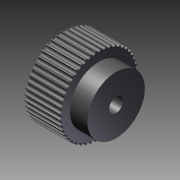
# Autodesk Inventor part: zrr_htd_3m15_8_17034800
Saved by Autodesk Inventor 2011 SP1 (Build 150282100, 282)
## iProperties
Created: 2018-07-07
Part Number: zrr_htd_3m15_8_17034800
Catalog Web Link: www.cadenas.de
Description: zrr_htd_3m15-HTD Pulleys Profile 3M, Timing Belt Width 15mm
Vendor: MAEDLER
Document SubType Name: Modeling
Designer: psAdmin
Manufacturer: MAEDLER
Mass: 101 g
Surface Area: 87.5363 cm^2
Volume: 36.8205 cm^3
Density: 1 g/cm^3
Category: PARTsolutions
Company: MAEDLER
Title: zrr_htd_3m15_8_17034800
Author: Cadenas PARTsolutions
Comments: HTD Pulleys Profile 3M, Timing Belt Width 15mm
PSOL_IDENT_0: {$CADENAS_DATA\23d-libs\maedler\antriebselemente\zahnriemenraeder_zahnriemen\zahnriemenraeder\htd-pr
PSOL_IDENT_1: ofil\zrr_htd_3m15.prj},197 {VTYP=3D},{NB=zrr_htd_3m15_8_17034800},{LINA=zrr_htd_3m15_8_17034800},{NN=
PSOL_IDENT_2: zrr_htd_3m15},{DATE=16.06.2017 10:47:49},{GEOMDATE=09.06.2016 09:07:07},{VERSION=},{LINEID=380},{LIN
PSOL_IDENT_3: ESUBID=-1},{WBVAR=BX}  {NB=zrr_htd_3m15_8_17034800},{LINA=zrr_htd_3m15_8_17034800},{KT=DUMMY},{ARTNR=
PSOL_IDENT_4: 17034800},{PDF=PDF Katalogseite},{AUSF=48-3M-15-2},{MAT=Aluminium},{ZTL=3.000},{ZRB=15.000},{Z=48.00
PSOL_IDENT_5: 0},{AUS=2},{ZS=45.080},{BS=0.000},{DO=45.840},{ND=33.000},{B=20.000},{L=30.000},{I=0.000},{VB=8.000}
PSOL_IDENT_6: ,{FB=20.000},{BX=8},{GEW=101.000},{ZT=1.200},{ZB=1.800},{T=2.000},{BB=1.000}
NN: zrr_htd_3m15
NT: HTD-Zahnriemenräder Profil 3M, Zahnriemenbreite 15mm
NB: zrr_htd_3m15_8_17034800
NBSYN: zrr_htd_3m15_$BX._$ARTNR.
LINA: zrr_htd_3m15_8_17034800
ARTNR: 17034800
PDF: PDF Katalogseite
AUSF: 48-3M-15-2
MAT: Aluminium
ZTL: 3.000
ZRB: 15.000
Z: 48.000
AUS: 2
ZS: 45.080
BS: 0.000
DO: 45.840
ND: 33.000
B: 20.000
L: 30.000
I: 0.000
VB: 8.000
FB: 20.000
BX: 8
GEW: 101.000
ZT: 1.200
ZB: 1.800
T: 2.000
BB: 1.000
SUPPLIER: MAEDLER
ARTICLENO: zrr_htd_3m15_8_17034800
BOMINFO: zrr_htd_3m15_8_17034800
CREATOR: CADENAS GmbH
Autodesk Inventor part; units mm, degrees
ref_plane "YZ Plane" through (0, 0, 0) normal (1, 0, 0) x (0, 1, 0)
ref_plane "XZ Plane" through (0, 0, 0) normal (0, 1, 0) x (-1, 0, 0)
ref_plane "XY Plane" through (0, 0, 0) normal (0, 0, 1) x (1, 0, 0)
sketch "Sketch_5" plane through (0, 0, 0) normal (0, 0, 1) x (1, 0, 0)
  line L0 (500, 0) -> (-500, 0)
  line L1 (0, 0) -> (0, 22.54)
  line L2 (0, 22.54) -> (20, 22.54)
  line L3 (20, 22.54) -> (20, 16.5)
  line L4 (20, 16.5) -> (30, 16.5)
  line L5 (30, 16.5) -> (30, 0)
  line L6 (30, 0) -> (0, 0)
  constraints: 14 end point
revolve "Revolution1" add sketch "Sketch_5" angle 360 about axis through (500, 0, 0) along (1, 0, 0)
sketch "Sketch_6" plane through (0, 0, 0) normal (1, 0, 0) x (0, 1, 0)
  circle A0 centre (0, 0) radius 300
  arc A1 (-1.1996, 22.5081) -> (1.1996, 22.5081) centre (0, 22.54) ccw
  arc A2 (-1.1996, 22.5081) -> (-1.4742, 22.4917) centre (0, 0) ccw
  arc A3 (-1.4742, 22.4917) -> (-1.7486, 22.4721) centre (0, 0) ccw
  arc A4 (-4.1272, 22.1589) -> (-1.7486, 22.4721) centre (-2.9421, 22.3472) ccw
  arc A5 (-4.1272, 22.1589) -> (-4.3973, 22.1069) centre (0, 0) ccw
  arc A6 (-4.3973, 22.1069) -> (-4.6668, 22.0516) centre (0, 0) ccw
  arc A7 (-6.9842, 21.4306) -> (-4.6668, 22.0516) centre (-5.8338, 21.772) ccw
  arc A8 (-6.9842, 21.4306) -> (-7.2452, 21.3438) centre (0, 0) ccw
  arc A9 (-7.2452, 21.3438) -> (-7.5052, 21.2538) centre (0, 0) ccw
  arc A10 (-9.7217, 20.3357) -> (-7.5052, 21.2538) centre (-8.6257, 20.8242) ccw
  arc A11 (-9.7217, 20.3357) -> (-9.9692, 20.2155) centre (0, 0) ccw
  arc A12 (-9.9692, 20.2155) -> (-10.2152, 20.0923) centre (0, 0) ccw
  arc A13 (-12.2929, 18.8928) -> (-10.2152, 20.0923) centre (-11.27, 19.5202) ccw
  arc A14 (-12.2929, 18.8928) -> (-12.5226, 18.7413) centre (0, 0) ccw
  arc A15 (-12.5226, 18.7413) -> (-12.7504, 18.5871) centre (0, 0) ccw
  arc A16 (-14.6537, 17.1266) -> (-12.7504, 18.5871) centre (-13.7215, 17.8822) ccw
  arc A17 (-14.6537, 17.1266) -> (-14.8617, 16.9465) centre (0, 0) ccw
  arc A18 (-14.8617, 16.9465) -> (-15.0674, 16.7638) centre (0, 0) ccw
  arc A19 (-16.7638, 15.0674) -> (-15.0674, 16.7638) centre (-15.9382, 15.9382) ccw
  arc A20 (-16.7638, 15.0674) -> (-16.9465, 14.8617) centre (0, 0) ccw
  arc A21 (-16.9465, 14.8617) -> (-17.1266, 14.6537) centre (0, 0) ccw
  arc A22 (-18.5871, 12.7504) -> (-17.1266, 14.6537) centre (-17.8822, 13.7215) ccw
  arc A23 (-18.5871, 12.7504) -> (-18.7413, 12.5226) centre (0, 0) ccw
  arc A24 (-18.7413, 12.5226) -> (-18.8928, 12.2929) centre (0, 0) ccw
  arc A25 (-20.0923, 10.2152) -> (-18.8928, 12.2929) centre (-19.5202, 11.27) ccw
  arc A26 (-20.0923, 10.2152) -> (-20.2155, 9.9692) centre (0, 0) ccw
  arc A27 (-20.2155, 9.9692) -> (-20.3357, 9.7217) centre (0, 0) ccw
  arc A28 (-21.2538, 7.5052) -> (-20.3357, 9.7217) centre (-20.8242, 8.6257) ccw
  arc A29 (-21.2538, 7.5052) -> (-21.3438, 7.2452) centre (0, 0) ccw
  arc A30 (-21.3438, 7.2452) -> (-21.4306, 6.9842) centre (0, 0) ccw
  arc A31 (-22.0516, 4.6668) -> (-21.4306, 6.9842) centre (-21.772, 5.8338) ccw
  arc A32 (-22.0516, 4.6668) -> (-22.1069, 4.3973) centre (0, 0) ccw
  arc A33 (-22.1069, 4.3973) -> (-22.1589, 4.1272) centre (0, 0) ccw
  arc A34 (-22.4721, 1.7486) -> (-22.1589, 4.1272) centre (-22.3472, 2.9421) ccw
  arc A35 (-22.4721, 1.7486) -> (-22.4917, 1.4742) centre (0, 0) ccw
  arc A36 (-22.4917, 1.4742) -> (-22.5081, 1.1996) centre (0, 0) ccw
  arc A37 (-22.5081, -1.1996) -> (-22.5081, 1.1996) centre (-22.54, 0) ccw
  arc A38 (-22.5081, -1.1996) -> (-22.4917, -1.4742) centre (0, 0) ccw
  arc A39 (-22.4917, -1.4742) -> (-22.4721, -1.7486) centre (0, 0) ccw
  arc A40 (-22.1589, -4.1272) -> (-22.4721, -1.7486) centre (-22.3472, -2.9421) ccw
  arc A41 (-22.1589, -4.1272) -> (-22.1069, -4.3973) centre (0, 0) ccw
  arc A42 (-22.1069, -4.3973) -> (-22.0516, -4.6668) centre (0, 0) ccw
  arc A43 (-21.4306, -6.9842) -> (-22.0516, -4.6668) centre (-21.772, -5.8338) ccw
  arc A44 (-21.4306, -6.9842) -> (-21.3438, -7.2452) centre (0, 0) ccw
  arc A45 (-21.3438, -7.2452) -> (-21.2538, -7.5052) centre (0, 0) ccw
  arc A46 (-20.3357, -9.7217) -> (-21.2538, -7.5052) centre (-20.8242, -8.6257) ccw
  arc A47 (-20.3357, -9.7217) -> (-20.2155, -9.9692) centre (0, 0) ccw
  arc A48 (-20.2155, -9.9692) -> (-20.0923, -10.2152) centre (0, 0) ccw
  arc A49 (-18.8928, -12.2929) -> (-20.0923, -10.2152) centre (-19.5202, -11.27) ccw
  arc A50 (-18.8928, -12.2929) -> (-18.7413, -12.5226) centre (0, 0) ccw
  arc A51 (-18.7413, -12.5226) -> (-18.5871, -12.7504) centre (0, 0) ccw
  arc A52 (-17.1266, -14.6537) -> (-18.5871, -12.7504) centre (-17.8822, -13.7215) ccw
  arc A53 (-17.1266, -14.6537) -> (-16.9465, -14.8617) centre (0, 0) ccw
  arc A54 (-16.9465, -14.8617) -> (-16.7638, -15.0674) centre (0, 0) ccw
  arc A55 (-15.0674, -16.7638) -> (-16.7638, -15.0674) centre (-15.9382, -15.9382) ccw
  arc A56 (-15.0674, -16.7638) -> (-14.8617, -16.9465) centre (0, 0) ccw
  arc A57 (-14.8617, -16.9465) -> (-14.6537, -17.1266) centre (0, 0) ccw
  arc A58 (-12.7504, -18.5871) -> (-14.6537, -17.1266) centre (-13.7215, -17.8822) ccw
  arc A59 (-12.7504, -18.5871) -> (-12.5226, -18.7413) centre (0, 0) ccw
  arc A60 (-12.5226, -18.7413) -> (-12.2929, -18.8928) centre (0, 0) ccw
  arc A61 (-10.2152, -20.0923) -> (-12.2929, -18.8928) centre (-11.27, -19.5202) ccw
  arc A62 (-10.2152, -20.0923) -> (-9.9692, -20.2155) centre (0, 0) ccw
  arc A63 (-9.9692, -20.2155) -> (-9.7217, -20.3357) centre (0, 0) ccw
  arc A64 (-7.5052, -21.2538) -> (-9.7217, -20.3357) centre (-8.6257, -20.8242) ccw
  arc A65 (-7.5052, -21.2538) -> (-7.2452, -21.3438) centre (0, 0) ccw
  arc A66 (-7.2452, -21.3438) -> (-6.9842, -21.4306) centre (0, 0) ccw
  arc A67 (-4.6668, -22.0516) -> (-6.9842, -21.4306) centre (-5.8338, -21.772) ccw
  arc A68 (-4.6668, -22.0516) -> (-4.3973, -22.1069) centre (0, 0) ccw
  arc A69 (-4.3973, -22.1069) -> (-4.1272, -22.1589) centre (0, 0) ccw
  arc A70 (-1.7486, -22.4721) -> (-4.1272, -22.1589) centre (-2.9421, -22.3472) ccw
  arc A71 (-1.7486, -22.4721) -> (-1.4742, -22.4917) centre (0, 0) ccw
  arc A72 (-1.4742, -22.4917) -> (-1.1996, -22.5081) centre (0, 0) ccw
  arc A73 (1.1996, -22.5081) -> (-1.1996, -22.5081) centre (0, -22.54) ccw
  arc A74 (1.1996, -22.5081) -> (1.4742, -22.4917) centre (0, 0) ccw
  arc A75 (1.4742, -22.4917) -> (1.7486, -22.4721) centre (0, 0) ccw
  arc A76 (4.1272, -22.1589) -> (1.7486, -22.4721) centre (2.9421, -22.3472) ccw
  arc A77 (4.1272, -22.1589) -> (4.3973, -22.1069) centre (0, 0) ccw
  arc A78 (4.3973, -22.1069) -> (4.6668, -22.0516) centre (0, 0) ccw
  arc A79 (6.9842, -21.4306) -> (4.6668, -22.0516) centre (5.8338, -21.772) ccw
  arc A80 (6.9842, -21.4306) -> (7.2452, -21.3438) centre (0, 0) ccw
  arc A81 (7.2452, -21.3438) -> (7.5052, -21.2538) centre (0, 0) ccw
  arc A82 (9.7217, -20.3357) -> (7.5052, -21.2538) centre (8.6257, -20.8242) ccw
  arc A83 (9.7217, -20.3357) -> (9.9692, -20.2155) centre (0, 0) ccw
  arc A84 (9.9692, -20.2155) -> (10.2152, -20.0923) centre (0, 0) ccw
  arc A85 (12.2929, -18.8928) -> (10.2152, -20.0923) centre (11.27, -19.5202) ccw
  arc A86 (12.2929, -18.8928) -> (12.5226, -18.7413) centre (0, 0) ccw
  arc A87 (12.5226, -18.7413) -> (12.7504, -18.5871) centre (0, 0) ccw
  arc A88 (14.6537, -17.1266) -> (12.7504, -18.5871) centre (13.7215, -17.8822) ccw
  arc A89 (14.6537, -17.1266) -> (14.8617, -16.9465) centre (0, 0) ccw
  arc A90 (14.8617, -16.9465) -> (15.0674, -16.7638) centre (0, 0) ccw
  arc A91 (16.7638, -15.0674) -> (15.0674, -16.7638) centre (15.9382, -15.9382) ccw
  arc A92 (16.7638, -15.0674) -> (16.9465, -14.8617) centre (0, 0) ccw
  arc A93 (16.9465, -14.8617) -> (17.1266, -14.6537) centre (0, 0) ccw
  arc A94 (18.5871, -12.7504) -> (17.1266, -14.6537) centre (17.8822, -13.7215) ccw
  arc A95 (18.5871, -12.7504) -> (18.7413, -12.5226) centre (0, 0) ccw
  arc A96 (18.7413, -12.5226) -> (18.8928, -12.2929) centre (0, 0) ccw
  arc A97 (20.0923, -10.2152) -> (18.8928, -12.2929) centre (19.5202, -11.27) ccw
  arc A98 (20.0923, -10.2152) -> (20.2155, -9.9692) centre (0, 0) ccw
  arc A99 (20.2155, -9.9692) -> (20.3357, -9.7217) centre (0, 0) ccw
  arc A100 (21.2538, -7.5052) -> (20.3357, -9.7217) centre (20.8242, -8.6257) ccw
  arc A101 (21.2538, -7.5052) -> (21.3438, -7.2452) centre (0, 0) ccw
  arc A102 (21.3438, -7.2452) -> (21.4306, -6.9842) centre (0, 0) ccw
  arc A103 (22.0516, -4.6668) -> (21.4306, -6.9842) centre (21.772, -5.8338) ccw
  arc A104 (22.0516, -4.6668) -> (22.1069, -4.3973) centre (0, 0) ccw
  arc A105 (22.1069, -4.3973) -> (22.1589, -4.1272) centre (0, 0) ccw
  arc A106 (22.4721, -1.7486) -> (22.1589, -4.1272) centre (22.3472, -2.9421) ccw
  arc A107 (22.4721, -1.7486) -> (22.4917, -1.4742) centre (0, 0) ccw
  arc A108 (22.4917, -1.4742) -> (22.5081, -1.1996) centre (0, 0) ccw
  arc A109 (22.5081, 1.1996) -> (22.5081, -1.1996) centre (22.54, 0) ccw
  arc A110 (22.5081, 1.1996) -> (22.4917, 1.4742) centre (0, 0) ccw
  arc A111 (22.4917, 1.4742) -> (22.4721, 1.7486) centre (0, 0) ccw
  arc A112 (22.1589, 4.1272) -> (22.4721, 1.7486) centre (22.3472, 2.9421) ccw
  arc A113 (22.1589, 4.1272) -> (22.1069, 4.3973) centre (0, 0) ccw
  arc A114 (22.1069, 4.3973) -> (22.0516, 4.6668) centre (0, 0) ccw
  arc A115 (21.4306, 6.9842) -> (22.0516, 4.6668) centre (21.772, 5.8338) ccw
  arc A116 (21.4306, 6.9842) -> (21.3438, 7.2452) centre (0, 0) ccw
  arc A117 (21.3438, 7.2452) -> (21.2538, 7.5052) centre (0, 0) ccw
  arc A118 (20.3357, 9.7217) -> (21.2538, 7.5052) centre (20.8242, 8.6257) ccw
  arc A119 (20.3357, 9.7217) -> (20.2155, 9.9692) centre (0, 0) ccw
  arc A120 (20.2155, 9.9692) -> (20.0923, 10.2152) centre (0, 0) ccw
  arc A121 (18.8928, 12.2929) -> (20.0923, 10.2152) centre (19.5202, 11.27) ccw
  arc A122 (18.8928, 12.2929) -> (18.7413, 12.5226) centre (0, 0) ccw
  arc A123 (18.7413, 12.5226) -> (18.5871, 12.7504) centre (0, 0) ccw
  arc A124 (17.1266, 14.6537) -> (18.5871, 12.7504) centre (17.8822, 13.7215) ccw
  arc A125 (17.1266, 14.6537) -> (16.9465, 14.8617) centre (0, 0) ccw
  arc A126 (16.9465, 14.8617) -> (16.7638, 15.0674) centre (0, 0) ccw
  arc A127 (15.0674, 16.7638) -> (16.7638, 15.0674) centre (15.9382, 15.9382) ccw
  arc A128 (15.0674, 16.7638) -> (14.8617, 16.9465) centre (0, 0) ccw
  arc A129 (14.8617, 16.9465) -> (14.6537, 17.1266) centre (0, 0) ccw
  arc A130 (12.7504, 18.5871) -> (14.6537, 17.1266) centre (13.7215, 17.8822) ccw
  arc A131 (12.7504, 18.5871) -> (12.5226, 18.7413) centre (0, 0) ccw
  arc A132 (12.5226, 18.7413) -> (12.2929, 18.8928) centre (0, 0) ccw
  arc A133 (10.2152, 20.0923) -> (12.2929, 18.8928) centre (11.27, 19.5202) ccw
  arc A134 (10.2152, 20.0923) -> (9.9692, 20.2155) centre (0, 0) ccw
  arc A135 (9.9692, 20.2155) -> (9.7217, 20.3357) centre (0, 0) ccw
  arc A136 (7.5052, 21.2538) -> (9.7217, 20.3357) centre (8.6257, 20.8242) ccw
  arc A137 (7.5052, 21.2538) -> (7.2452, 21.3438) centre (0, 0) ccw
  arc A138 (7.2452, 21.3438) -> (6.9842, 21.4306) centre (0, 0) ccw
  arc A139 (4.6668, 22.0516) -> (6.9842, 21.4306) centre (5.8338, 21.772) ccw
  arc A140 (4.6668, 22.0516) -> (4.3973, 22.1069) centre (0, 0) ccw
  arc A141 (4.3973, 22.1069) -> (4.1272, 22.1589) centre (0, 0) ccw
  arc A142 (1.7486, 22.4721) -> (4.1272, 22.1589) centre (2.9421, 22.3472) ccw
  arc A143 (1.7486, 22.4721) -> (1.4742, 22.4917) centre (0, 0) ccw
  arc A144 (1.4742, 22.4917) -> (1.1996, 22.5081) centre (0, 0) ccw
  constraints: 288 point on circle, 145 centre point
extrude "Extrusion1" cut sketch "Sketch_6" along normal blind 20
sketch "Sketch_9_ALT_Drilling_1" plane through (0, 0, 0) normal (1, 0, 0) x (0, 1, 0)
  circle A0 centre (0, 0) radius 4
  constraints: 1 centre point
extrude "Extrusion2" cut sketch "Sketch_9_ALT_Drilling_1" along normal blind 30
body "Solid1"
